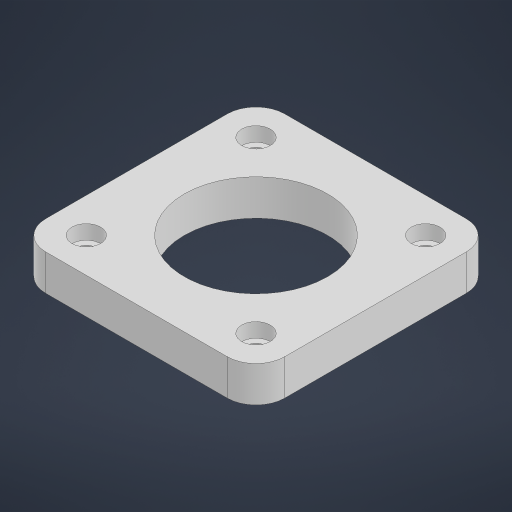
# Autodesk Inventor part: CamTest2
Saved by Autodesk Inventor 2024.2 (Build 282272000, 272)
## iProperties
Created: 2024-04-15
Part Number: CamTest2
Material: Generic
Document SubType Name: Modeling
Designer: fablabadmin
Density: 1 g/cm^3
Appearance: Default
Author: fablabadmin
Autodesk Inventor part; units mm, degrees
ref_plane "YZ Plane" through (0, 0, 0) normal (1, 0, 0) x (0, 1, 0)
ref_plane "XZ Plane" through (0, 0, 0) normal (0, 1, 0) x (-1, 0, 0)
ref_plane "XY Plane" through (0, 0, 0) normal (0, 0, 1) x (1, 0, 0)
sketch "Sketch1" plane through (0, 0, 0) normal (0, 1, 0) x (-1, 0, 0)
  line L0 (-50, 50) -> (50, 50)
  line L1 (50, 50) -> (50, -50)
  line L2 (50, -50) -> (-50, -50)
  line L3 (-50, -50) -> (-50, 50)
  line L4 (-50, 50) -> (50, -50) construction
  line L5 (50, 50) -> (-50, -50) construction
  line L6 (-35.5, 35.5) -> (35.5, 35.5) construction
  line L7 (35.5, 35.5) -> (35.5, -35.5) construction
  line L8 (35.5, -35.5) -> (-35.5, -35.5) construction
  line L9 (-35.5, -35.5) -> (-35.5, 35.5) construction
  line L10 (-35.5, 35.5) -> (35.5, -35.5) construction
  line L11 (35.5, 35.5) -> (-35.5, -35.5) construction
  circle A0 centre (0, 0) radius 30
  dimension "d0" = 100
  dimension "d1" = 71
  dimension "d2" = 60
  constraints: 24 end point, 4 coincident, 4 midpoint, 4 parallel, 3 perpendicular, 2 horizontal, 1 centre point, 1 point on line
  measures "d0" distance of L1.end L2.end
  measures "d1" distance of L7.end L8.end
  measures "d2" diameter of A0
extrude "Extrusion1" add sketch "Sketch1" against normal blind 15
hole "Hole1" at (-35.5, 0, -35.5) at (35.5, 0, -35.5) at (-35.5, 0, 35.5) at (35.5, 0, 35.5) direction (0, -1, 0) diameter 7 end through all counterbore diameter 12 counterbore depth 6
fillet "Fillet1" radius 12 4 edges at (-50, -7.5, 50) (-50, -7.5, -50) (50, -7.5, -50) (50, -7.5, 50)
body "Solid1"
